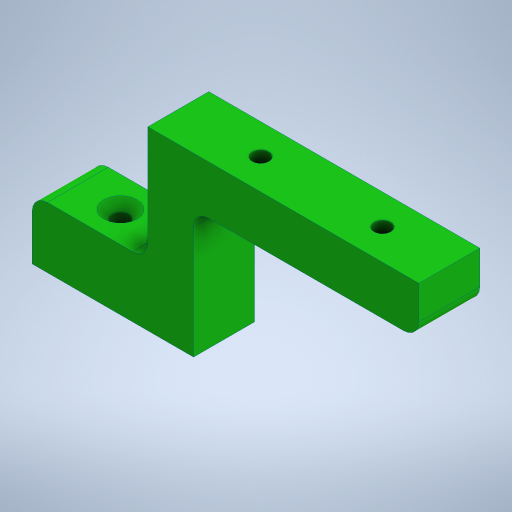
# Autodesk Inventor part: unión placa soporte TIC DC
Saved by Autodesk Inventor 2024.2 (Build 282272000, 272)
## iProperties
Created: 2024-08-28
Part Number: unión placa soporte TIC DC
Material: PET Plastic
Document SubType Name: Modeling
Designer: ja.restrepo1
Density: 1.541 g/cm^3
Appearance: Sky Blue Dark
Author: ja.restrepo1
Autodesk Inventor part; units mm, degrees
ref_plane "YZ Plane" through (0, 0, 0) normal (1, 0, 0) x (0, 1, 0)
ref_plane "XZ Plane" through (0, 0, 0) normal (0, 1, 0) x (-1, 0, 0)
ref_plane "XY Plane" through (0, 0, 0) normal (0, 0, 1) x (1, 0, 0)
sketch "Sketch1" plane through (0, 0, 0) normal (0, 0, 1) x (1, 0, 0)
  line L0 (-89, 58) -> (0, 58)
  line L1 (0, 42) -> (-74, 42)
  line L2 (-74, 42) -> (-74, 0)
  line L3 (-74, 0) -> (-127, 0)
  line L4 (-127, 0) -> (-127, 20)
  line L5 (-127, 20) -> (-89, 20)
  line L6 (-89, 20) -> (-89, 58)
  line L7 (0, 58) -> (0, 42)
  point P0 (0, 0)
  point P1 (0, 50)
  point P2 (-100.5, 0)
  dimension "d116" = 15
  dimension "d128" = 89
  dimension "d129" = 16
  dimension "d130" = 20
  dimension "d131" = 53
  dimension "d132" = 38
  dimension "d135" = 74
  constraints: 16 end point, 4 perpendicular, 2 midpoint, 2 vertical, 1 horizontal, 1 horizontal alignment, 1 vertical alignment
  measures "d116" distance between parallel lines of L6 L2
  measures "d128" distance of L0.start L0.end
  measures "d129" distance between parallel lines of L0 L1
  measures "d130" distance between parallel lines of L3 L5
  measures "d131" distance of L2.end L3.end
  measures "d132" distance between parallel lines of L0 L5
  measures "d135" distance of L1.start L1.end
extrude "Soporte" add sketch "Sketch1" along normal mid plane 20
sketch "Sketch13" plane through (-74, 42, 10) normal (0, 1, 0) x (1, 0, 0)
  line L0 (12, 10) -> (52, 10) construction
  line L1 (0, 20) -> (0, 0) projected
  line L2 (0, 0) -> (74, 0) projected
  point P0 (74, 10)
  point P1 (32, 10)
  point P2 (-15, 20)
  point P3 (74, 20)
  point P4 (0, 10)
  dimension "d104" = 40
  dimension "d133" = 32
  constraints: 2 end point, 2 midpoint, 1 horizontal, 1 horizontal alignment
  measures "d104" distance of L0.start L0.end
  measures "d133" distance from line of point (32, 10) L1
hole "BCA M5" at (-62, 42, 0) at (-22, 42, 0) direction (0, 1, 0) diameter 5.5 end through all countersink diameter 11 countersink angle 90
fillet "Fillet7" radius 5 4 edges at (-89, 20, 0) (-74, 42, 0) (-127, 20, 0) (0, 42, 0)
sketch "Sketch15" plane through (-122, 20, 10) normal (0, 1, 0) x (1, 0, 0)
  line L0 (28, 0) -> (0, 0) projected
  line L1 (0, 0) -> (0, 20) projected
  point P0 (122, 10)
  point P1 (14, 10)
  point P2 (14, 0)
  point P3 (0, 10)
  constraints: 2 midpoint, 1 horizontal alignment, 1 vertical alignment
hole "Hole8" at (-108, 20, 0) direction (0, -1, 0) diameter 5.5 end through all countersink diameter 11 countersink angle 90
body "Solid1"
